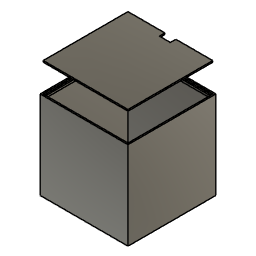
NoteBlockMaestro (Autodesk Fusion 360 design; units mm, degrees)
part number: 2025-07-01-10-41-04-519
Autodesk Fusion 360 part; units mm, degrees
sketch "Sketch1" plane through (0, 0, 0) normal (0, 0, 1) x (1, 0, 0)
  line L0 (0, 0) -> (152, 0)
  line L1 (152, 0) -> (152, -152)
  line L2 (152, -152) -> (0, -152)
  line L3 (0, -152) -> (0, 0)
  dimension "d1" = 152
  dimension "d2" = 152
  constraint horizontal L0
  constraint vertical L1
  constraint horizontal L2
  constraint vertical L3
  constraint coincident L0.start L3.end
  measures "d1" distance of L0.start L0.end
  measures "d2" distance of L0.start L2.end
extrude "Extrude1" add sketch "Sketch1" along normal blind 152 makes body 1
move_body "Move1" bodies 1 to x (1, 0, 0) y (0, 1, 0) z (0, 0, 1) at (76, 0, 0)
move_body "Move2" bodies 1 to x (1, 0, 0) y (0, 1, 0) z (0, 0, 1) at (-152, 0, 0)
move_body "Move3" bodies 1 to x (1, 0, 0) y (0, 1, 0) z (0, 0, 1) at (0, -76, 0)
move_body "Move4" bodies 1 to x (1, 0, 0) y (0, 1, 0) z (0, 0, 1) at (0, 152, 0)
shell "Shell1" thickness 2.5 removed faces 1 at (-25.3333, 25.3333, 152) on bodies 1
sketch "Sketch2" plane through (0, 0, 152) normal (0, 0, 1) x (-1, 0, 0)
  line L0 (73.5, 73.5) -> (73.5, -73.5)
  line L1 (73.5, -73.5) -> (-73.5, -73.5)
  line L2 (-73.5, -73.5) -> (-73.5, 73.5)
  line L3 (-73.5, 73.5) -> (73.5, 73.5)
  line L4 (76, 76) -> (-76, 76)
  line L5 (-76, 76) -> (-76, -76)
  line L6 (-76, -76) -> (76, -76)
  line L7 (76, -76) -> (76, 76)
  line L8 (76, -76) -> (-76, -76)
  line L9 (-76, -76) -> (-76, 76)
  line L10 (-76, 76) -> (76, 76)
  line L11 (76, 76) -> (76, -76)
  constraint horizontal L8
  constraint vertical L9
  constraint horizontal L10
  constraint vertical L11
  constraint coincident L4.end L5.start
  constraint coincident L6.end L7.start
extrude "Extrude2" add sketch "Sketch2" along normal blind 2.5 separate body contours L0 L1 L2 L3 makes body 2
move_body "Move5" bodies 2 to x (1, 0, 0) y (0, 1, 0) z (0, 0, 1) at (0, 0, 100)
ref_plane "WorkPlane1" through (0, 0, 149.5) normal (0, 0, 1) x (1, 0, 0)
sketch "Sketch3" plane through (0, 0, 149.5) normal (0, 0, 1) x (1, 0, 0)
  line L0 (73.5, 73.5) -> (-73.5, 73.5)
  line L1 (-73.5, 73.5) -> (-73.5, -73.5)
  line L2 (-73.5, -73.5) -> (73.5, -73.5)
  line L3 (73.5, -73.5) -> (73.5, 73.5)
  line L4 (-72.5, -72.5) -> (72.5, -72.5)
  line L5 (72.5, -72.5) -> (72.5, 72.5)
  line L6 (72.5, 72.5) -> (-72.5, 72.5)
  line L7 (-72.5, 72.5) -> (-72.5, -72.5)
  point P0 (-73.5, 73.5)
  point P1 (73.5, 73.5)
  point P2 (-73.5, -73.5)
  point P3 (73.5, -73.5)
  dimension "d9" = -1
  constraint horizontal L0
  constraint vertical L1
  constraint horizontal L2
  constraint vertical L3
  constraint coincident P2 L1.end
  constraint coincident P1 L0.start
extrude "Extrude3" add sketch "Sketch3" against normal blind 2 bodies 1
extrude "Extrude4" add 1 faces at (-72.5, 24.1667, 148.8333) along direction (1, 0, 0) blind 1 on bodies 1 bodies 1
extrude "Extrude5" add 1 faces at (24.5, 72.5, 148.8333) along direction (0, -1, 0) blind 1 on bodies 1 bodies 1
extrude "Extrude6" add 1 faces at (72.5, -24.5, 148.8333) along direction (-1, 0, 0) blind 1 on bodies 1 bodies 1
extrude "Extrude7" add 1 faces at (-23.8333, -72.5, 148.1667) along direction (0, 1, 0) blind 1 on bodies 1 bodies 1
extrude "Extrude8" add 1 faces at (-73.5, -24.5, 252.8333) along direction (-1, 0, 0) blind 0.1 on bodies 2 bodies 2
extrude "Extrude9" cut 1 faces at (-73.6, -24.5, 252.8333) along direction (1, 0, 0) blind 0.2 on bodies 2 bodies 2
extrude "Extrude10" cut 1 faces at (24.5333, -73.5, 252.8333) along direction (0, 1, 0) blind 0.2 on bodies 2 bodies 2
extrude "Extrude11" cut 1 faces at (73.5, 24.5667, 252.8333) along direction (-1, 0, 0) blind 0.2 on bodies 2 bodies 2
extrude "Extrude12" cut 1 faces at (-24.5, 73.5, 253.6667) along direction (0, -1, 0) blind 0.2 on bodies 2 bodies 2
move_body "Move6" bodies 2 to x (1, 0, 0) y (0, 1, 0) z (0, 0, 1) at (0, 0, -60)
sketch "Sketch4" plane through (0, 0, 194.5) normal (0, 0, 1) x (-1, 0, 0)
  line L0 (-73.3, -73.3) -> (73.4, -73.3)
  line L1 (73.4, -73.3) -> (73.4, 73.3)
  line L2 (73.4, 73.3) -> (-73.3, 73.3)
  line L3 (-73.3, 73.3) -> (-73.3, -73.3)
  line L4 (0.05, -73.3) -> (9.55, -73.3)
  line L5 (0.05, -73.3) -> (-9.45, -73.3)
  line L6 (-9.45, -73.3) -> (-9.45, -63.8)
  line L7 (-9.45, -63.8) -> (0.05, -63.8)
  line L8 (0.05, -63.8) -> (9.55, -63.8)
  line L9 (9.55, -63.8) -> (9.55, -73.3)
  dimension "d30" = 9.5
  dimension "d31" = 9.5
  dimension "d32" = 9.5
  dimension "d33" = 9.5
  dimension "d34" = 9.5
  dimension "d35" = 9.5
  constraint midpoint L0 L4.start
  constraint parallel L0 L4
  constraint parallel L0 L5
  constraint perpendicular L5 L6
  constraint perpendicular L6 L7
  constraint perpendicular L6 L8
  constraint perpendicular L4 L9
  measures "d30" distance of L4.start L4.end
  measures "d31" distance of L4.start L5.end
  measures "d32" distance of L5.end L6.end
  measures "d33" distance of L6.end L7.end
  measures "d34" distance of L7.end L8.end
  measures "d35" distance of L8.end L4.end
extrude "Extrude13" cut sketch "Sketch4" against normal blind 2.5 contours L0 L4 L5 L6 L7 L8 L9 bodies 2
move_body "Move7" bodies 2 to x (1, 0, 0) y (0, 1, 0) z (0, 0, 1) at (0, 0, -42.5)
sketch "Sketch5" plane through (0, 0, 149.5) normal (0, 0, 1) x (-1, 0, 0)
  line L0 (71.5, 71.5) -> (71.5, -71.5)
  line L1 (71.5, -71.5) -> (-71.5, -71.5)
  line L2 (-71.5, -71.5) -> (-71.5, 71.5)
  line L3 (-71.5, 71.5) -> (71.5, 71.5)
  line L4 (-73.5, 73.5) -> (-73.5, -73.5)
  line L5 (-73.5, -73.5) -> (73.5, -73.5)
  line L6 (73.5, -73.5) -> (73.5, 73.5)
  line L7 (73.5, 73.5) -> (-73.5, 73.5)
  line L8 (9.55, -73.5) -> (-9.4425, -73.5)
  line L9 (-9.4425, -73.5) -> (-9.4425, -71.5)
  line L10 (-9.4425, -71.5) -> (9.55, -71.5)
  line L11 (9.55, -71.5) -> (9.55, -73.5)
  constraint horizontal L8
  constraint vertical L9
  constraint horizontal L10
  constraint vertical L11
  constraint coincident L1 L9.end
  constraint coincident L5 L8.start
extrude "Extrude14" cut sketch "Sketch5" against normal blind 2 contours L1 L5 L8 L9 L10 L11 bodies 1
move_body "Move8" bodies 2 to x (1, 0, 0) y (0, 1, 0) z (0, 0, 1) at (0, 0, 50)
extrude "Extrude15" add 1 faces at (71.5, -23.8333, 148.1667) along direction (-1, 0, 0) blind 0.5 on bodies 1 bodies 1
extrude "Extrude16" add 1 faces at (50.4808, 71.5, 148.8333) along direction (0, -1, 0) blind 0.5 on bodies 1 bodies 1
extrude "Extrude17" add 1 faces at (-71.5, 23.8333, 148.1667) along direction (1, 0, 0) blind 0.5 on bodies 1 bodies 1
extrude "Extrude18" add 1 faces at (-23.6667, -71.5, 148.8333) along direction (0, 1, 0) blind 0.5 on bodies 1 bodies 1
extrude "Extrude19" add 1 faces at (-23.6667, -72.6667, 147.5) along direction (0, 0, -1) blind 0.5 on bodies 1 bodies 1
extrude "Extrude20" add 1 faces at (-23.6667, -72.6667, 147) along direction (0, 0, -1) blind 1 on bodies 1 bodies 1
scale "Scale1" factor 1.157895 about (71, -71, 146) bodies 1 2
equation "d52 = 22 / 19"
